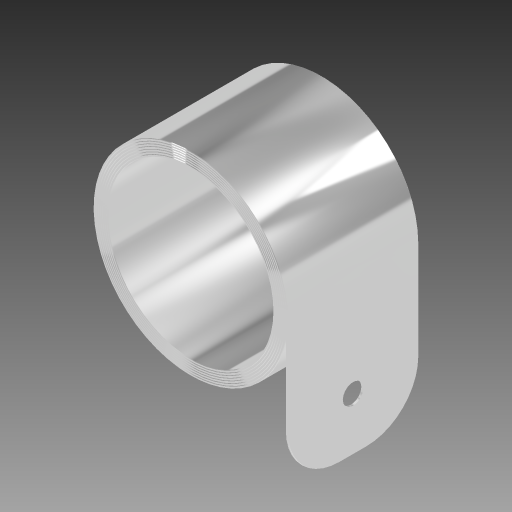
# Autodesk Inventor part: TTB Elevator Constant Force Spring
Saved by Autodesk Inventor 2023 (Build 270158000, 158)
## iProperties
Created: 2023-01-02
Part Number: TTB Elevator Constant Force Spring
Material: Steel
Document SubType Name: Modeling
Designer: Max Boord
Mass: 122.831 g
Surface Area: 115.939 cm^2
Volume: 15.6473 cm^3
Density: 7.85 g/cm^3
Appearance: Chrome - Polished
Author: Max Boord
Autodesk Inventor part; units mm, degrees
ref_plane "YZ Plane" through (0, 0, 0) normal (1, 0, 0) x (0, 1, 0)
ref_plane "XZ Plane" through (0, 0, 0) normal (0, 1, 0) x (-1, 0, 0)
ref_plane "XY Plane" through (0, 0, 0) normal (0, 0, 1) x (1, 0, 0)
sketch "Sketch1" plane through (0, 0, 0) normal (0, 0, 1) x (1, 0, 0)
  circle A0 centre (0, 0) radius 20
  circle A1 centre (0, 0) radius 23.5
  line L0 (23.5, 0) -> (23, 0)
  line L1 (23, 0) -> (23, -36.2)
  line L2 (23, -36.2) -> (23.5, -36.2)
  line L3 (23.5, -36.2) -> (23.5, 0)
  circle A2 centre (0, 0) radius 23
  circle A3 centre (0, 0) radius 22.5
  circle A4 centre (0, 0) radius 22
  circle A5 centre (0, 0) radius 21.5
  circle A6 centre (0, 0) radius 21
  circle A7 centre (0, 0) radius 20.5
  point P0 (23, -4.8218)
  point P1 (0, -23.5)
  dimension "d0" = 40
  dimension "d1" = 47
  dimension "d2" = 0.5
  dimension "d3" = 0.5
  dimension "d4" = 0.5
  dimension "d5" = 0.5
  dimension "d6" = 0.5
  dimension "d7" = 0.5
  dimension "d58" = 12.7
  constraints: 8 end point, 7 centre point, 4 coincident, 2 horizontal alignment, 2 parallel, 2 point on circle, 1 horizontal, 1 perpendicular, 1 vertical alignment, 2 other
  measures "d0" diameter of A0
  measures "d1" diameter of A1
  measures "d2" distance between parallel lines of L3 L1
  measures "d4" radial gap between concentric circles of A3 A4
  measures "d5" radial gap between concentric circles of A4 A5
  measures "d6" radial gap between concentric circles of A5 A6
  measures "d7" radial gap between concentric circles of A6 A7
  measures "d58" distance from line of L2 A1.end
extrude "Extrusion1" add sketch "Sketch1" along normal mid plane 31.75 contours A7
chamfer "Chamfer3" distance 0.1 angle 45 4 edges at (-20.5, 0, 15.875) (-20, 0, 15.875) (-20.5, 0, -15.875) (-20, 0, -15.875)
extrude "Extrusion2" add sketch "Sketch1" along normal mid plane 31.75 contours A6
chamfer "Chamfer4" distance 0.1 angle 45 4 edges at (-21, 0, 15.875) (-21, 0, -15.875) (-20.5, 0, 15.875) (-20.5, 0, -15.775)
extrude "Extrusion3" add sketch "Sketch1" along normal mid plane 31.75 contours A5
chamfer "Chamfer5" distance 0.1 angle 45 4 edges at (-21.5, 0, 15.875) (-21, 0, 15.875) (-21.5, 0, -15.875) (-21, 0, -15.875)
extrude "Extrusion4" add sketch "Sketch1" along normal mid plane 31.75 contours A4
chamfer "Chamfer6" distance 0.1 angle 45 4 edges at (-22, 0, 15.875) (-21.5, 0, 15.875) (-22, 0, -15.875) (-21.5, 0, -15.875)
extrude "Extrusion5" add sketch "Sketch1" along normal mid plane 31.75 contours A3
chamfer "Chamfer7" distance 0.1 angle 45 4 edges at (-22.5, 0, 15.875) (-22, 0, 15.875) (-22.5, 0, -15.875) (-22, 0, -15.875)
extrude "Extrusion6" add sketch "Sketch1" along normal mid plane 31.75 contours A2
chamfer "Chamfer8" distance 0.1 angle 45 4 edges at (-23, 0, 15.875) (-22.5, 0, 15.875) (-23, 0, -15.875) (-22.5, 0, -15.875)
extrude "Extrusion7" add sketch "Sketch1" along normal mid plane 31.75 contours L0 L1 A1 | L3 L2 L1 A1 | A1 L1 L0
fillet "Fillet1" radius 12.7 2 edges at (23.25, -36.2, 15.875) (23.25, -36.2, -15.875)
chamfer "Chamfer9" distance 0.1 angle 45 9 edges at (23.5, -11.75, 15.875) (-23.3747, 2.4238, 15.875) (23.5, -32.4803, 12.1553) (23.5, -11.75, -15.875) (-23.3747, 2.4238, -15.875) (-23, 0, 15.875) (23, -14.1609, 15.875) (23, -32.4803, 12.1553) (23, -14.1609, -15.875)
sketch "Sketch2" plane through (23.5, -23.5, 15.775) normal (1, 0, 0) x (0, 0, -1)
  line L0 (0, 0) -> (0, 23.5) projected
  arc A0 (0, 0) -> (12.6, -12.6) centre (12.6, 0) ccw projected
  line L1 (18.95, -12.6) -> (12.6, -12.6) projected
  arc A1 (18.95, -12.6) -> (31.55, 0) centre (18.95, 0) ccw projected
  line L2 (31.55, 23.5) -> (31.55, 0) projected
  line L3 (31.55, 23.5) -> (0, 23.5) projected
  line L4 (12.6, 0) -> (18.95, 0)
  point P0 (15.775, 23.5)
  point P1 (15.775, 0)
  constraints: 2 end point, 1 horizontal, 1 midpoint
hole "Hole1" at (23.5, -23.5, 0) direction (-1, 0, 0) diameter 4.9784 depth 0.5 tip angle 118
equation "\"d3\" = d2"
equation "\"d13\" = Thickness"
equation "\"d18\" = Thickness"
equation "\"d20\" = Thickness"
equation "\"d22\" = Thickness"
equation "\"d24\" = Thickness"
equation "\"d26\" = Thickness"
equation "\"Thickness\" = 31.75"
body "Solid1"
